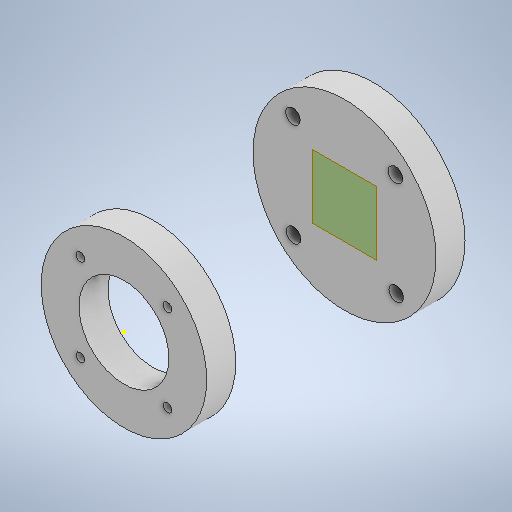
# Autodesk Inventor part: LightBracket
Saved by Autodesk Inventor 2025.2 (Build 292293000, 293)
## iProperties
Created: 2025-03-20
Part Number: LightBracket
Material: Generic
Document SubType Name: Modeling
Designer: Victor
Density: 1 g/cm^3
Appearance: Default
Author: Victor
Autodesk Inventor part; units mm, degrees
ref_plane "YZ Plane" through (0, 0, 0) normal (1, 0, 0) x (0, 1, 0)
ref_plane "XZ Plane" through (0, 0, 0) normal (0, 1, 0) x (-1, 0, 0)
ref_plane "XY Plane" through (0, 0, 0) normal (0, 0, 1) x (1, 0, 0)
sketch "Sketch1" plane through (0, 0, 0) normal (0, 0, 1) x (1, 0, 0)
  circle A0 centre (0, 0) radius 28.5
  circle A1 centre (0, 0) radius 15.5
  circle A2 centre (-15, 15) radius 1.5
  circle A3 centre (15, 15) radius 1.5
  circle A4 centre (15, -15) radius 1.5
  circle A5 centre (-15, -15) radius 1.5
  dimension "d0" = 57
  dimension "d1" = 31
  dimension "d6" = 3
  dimension "d7" = 3
  dimension "d8" = 3
  dimension "d9" = 3
  constraints: 6 centre point, 3 coincident
  measures "d0" diameter of A0
  measures "d1" diameter of A1
  measures "d6" diameter of A2
  measures "d7" diameter of A3
  measures "d8" diameter of A4
  measures "d9" diameter of A5
extrude "Extrusion1" add sketch "Sketch1" along normal blind 10
ref_plane "Work Plane14" through (0, 0, -66) normal (0, 0, -1) x (-1, 0, 0)
sketch "Sketch2" plane through (0, 0, -66) normal (0, 0, -1) x (-1, 0, 0)
  circle A0 centre (0, 0) radius 31.5
  circle A1 centre (0, 0) radius 16.75
  circle A2 centre (17.7849, 17.5698) radius 2.5
  circle A3 centre (-17.5698, 17.7849) radius 2.5
  circle A4 centre (-17.7849, -17.5698) radius 2.5
  circle A5 centre (17.5698, -17.7849) radius 2.5
  dimension "d13" = 63
  dimension "d14" = 33.5
  dimension "d16" = 5
  dimension "d19" = 360
  constraints: 6 centre point, 3 coincident, 9 other
  measures "d13" diameter of A0
  measures "d14" diameter of A1
  measures "d16" diameter of A2
extrude "Extrusion2" add sketch "Sketch2" along normal blind 10
sketch "Sketch3" plane through (0, 0, 10) normal (0, 0, 1) x (1, 0, 0)
  point P0 (0, 0)
ref_plane "Work Plane28" through (0, 0, -66) normal (0, 0, -1) x (-1, 0, 0)
sketch "Sketch4" plane through (0, 0, -66) normal (0, 0, -1) x (-1, 0, 0)
  circle A0 centre (0, 0) radius 16.75
  dimension "d23" = 33.5
  constraints: 1 centre point, 1 coincident
  measures "d23" diameter of A0
extrude "Extrusion3" add sketch "Sketch4" along normal blind 10
ref_plane "Work Plane27" through (0, 0, -76) normal (0, 0, -1) x (-1, 0, 0)
sketch "Sketch5" plane through (0, 0, -76) normal (0, 0, -1) x (-1, 0, 0)
  circle A0 centre (0, 0) radius 15.5
  dimension "d26" = 31
  constraints: 1 centre point, 1 coincident
  measures "d26" diameter of A0
extrude "Extrusion4" add sketch "Sketch5" along normal blind 5
sketch "Sketch12" plane through (0, 0, 10) normal (0, 0, 1) x (1, 0, 0)
  point P0 (0, 0)
body "Solid1"
